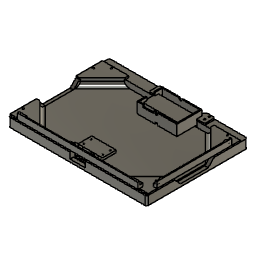
fusion_export (Autodesk Fusion 360 design; units mm, degrees)
Autodesk Fusion 360 part; units mm, degrees
note: some values were not read from the file. Chosen so that the rebuilt part matches the saved one: which face or edge a step refers to. Set by a fixed rule: which sketch regions a step uses.
sketch "Skizze1" plane through (0, 0, 0) normal (0, 0, 1) x (1, 0, 0)
  line L0 (88.5, 66) -> (-88.5, 66)
  line L1 (-90.5, 64) -> (-90.5, -64)
  line L2 (-88.5, -66) -> (88.5, -66)
  line L3 (90.5, -64) -> (90.5, 64)
  line L4 (90.5, 66) -> (-90.5, -66) construction
  line L5 (-90.5, 66) -> (90.5, -66) construction
  line L6 (-86, 52.5) -> (86, 52.5)
  line L7 (86, 52.5) -> (86, -59.5)
  line L8 (86, -59.5) -> (-86, -59.5)
  line L9 (-86, -59.5) -> (-86, 52.5)
  line L10 (0, 0) -> (0, 110) construction
  line L11 (-74, 48.5) -> (74, 48.5)
  line L12 (74, 48.5) -> (74, -48.5)
  line L13 (74, -48.5) -> (-74, -48.5)
  line L14 (-74, -48.5) -> (-74, 48.5)
  line L15 (0, 0) -> (180, 0) construction
  line L16 (-10, -59.5) -> (10, -59.5)
  line L17 (10, -59.5) -> (10, -66)
  line L18 (10, -66) -> (-10, -66)
  line L19 (-10, -66) -> (-10, -59.5)
  arc A0 (-90.5, -64) -> (-88.5, -66) centre (-88.5, -64) ccw
  arc A1 (88.5, -66) -> (90.5, -64) centre (88.5, -64) ccw
  arc A2 (-88.5, 66) -> (-90.5, 64) centre (-88.5, 64) ccw
  arc A3 (90.5, 64) -> (88.5, 66) centre (88.5, 64) ccw
  circle A4 centre (-12.5, -62) radius 0.9
  circle A5 centre (12.5, -62) radius 0.9
  line L20 (-20, -66) -> (-20, -59.5)
  line L21 (20, -59.5) -> (20, -66)
  circle A6 centre (-88, -49.5) radius 0.9
  circle A7 centre (-76, -61.5) radius 0.9
  line L22 (130, -3.5) -> (-113.5332, -3.5) construction
  line L23 (-86, -29.5) -> (-90.5, -29.5)
  line L24 (-56, -59.5) -> (-56, -66)
  line L25 (86, -29.5) -> (90.5, -29.5)
  circle A8 centre (88, -49.5) radius 0.9
  circle A9 centre (76, -61.5) radius 0.9
  line L26 (56, -59.5) -> (56, -66)
  line L27 (-86, 22.5) -> (-90.5, 22.5)
  circle A10 centre (-76, 54.5) radius 0.9
  line L28 (-56, 52.5) -> (-56, 59)
  line L29 (56, 52.5) -> (56, 59)
  line L30 (86, 22.5) -> (90.5, 22.5)
  circle A11 centre (76, 54.5) radius 0.9
  circle A12 centre (88, 42.5) radius 0.9
  circle A13 centre (-88, 42.5) radius 0.9
  line L31 (-56, 59) -> (-90.5, 59)
  line L32 (56, 59) -> (90.5, 59)
  line L33 (-56, 52.5) -> (-86, 22.5)
  line L34 (56, 52.5) -> (86, 22.5)
  line L35 (-86, -29.5) -> (-56, -59.5)
  line L36 (86, -29.5) -> (56, -59.5)
  line L37 (-56, -64) -> (-90.5, -64)
  line L38 (56, -64) -> (90.5, -64)
  line L39 (56, 57) -> (90.5, 57)
  line L40 (-56, 57) -> (-90.5, 57)
  line L41 (-13, 58) -> (36, 58)
  line L42 (36, 58) -> (36, 28)
  line L43 (36, 28) -> (-13, 28)
  line L44 (-13, 28) -> (-13, 58)
  line L45 (-14.5, 26.5) -> (-14.5, 59.5)
  line L46 (-14.5, 59.5) -> (37.5, 59.5)
  line L47 (37.5, 59.5) -> (37.5, 26.5)
  line L48 (37.5, 26.5) -> (-14.5, 26.5)
  line L49 (-7, 28) -> (7, 28)
  line L50 (7, 28) -> (7, 26.5)
  line L51 (7, 26.5) -> (-7, 26.5)
  line L52 (-7, 26.5) -> (-7, 28)
  line L53 (-14.5, 48) -> (-13, 48)
  line L54 (-13, 48) -> (-13, 38)
  line L55 (-13, 38) -> (-14.5, 38)
  line L56 (-14.5, 38) -> (-14.5, 48)
  line L57 (41, 43) -> (-35, 43) construction
  circle A14 centre (-20, 54.5) radius 0.9
  circle A15 centre (43, 54.5) radius 0.9
  line L58 (-25, 52.5) -> (-15, 52.5)
  line L59 (-15, 52.5) -> (-15, 66)
  line L60 (-15, 66) -> (-25, 66)
  line L61 (-25, 66) -> (-25, 52.5)
  line L62 (48, 52.5) -> (38, 52.5)
  line L63 (38, 52.5) -> (38, 66)
  line L64 (38, 66) -> (48, 66)
  line L65 (48, 66) -> (48, 52.5)
  line L66 (76, 54.5) -> (-76, 54.5) construction
  circle A16 centre (43, 57.5) radius 0.9
  circle A17 centre (-20, 57.5) radius 0.9
  circle A18 centre (43, 60.5) radius 0.9
  circle A19 centre (-20, 60.5) radius 0.9
  circle A20 centre (43, 63.5) radius 0.9
  circle A21 centre (-20, 63.5) radius 0.9
  line L67 (-16, -66) -> (16, -66)
  line L68 (16, -66) -> (16, -31.5)
  line L69 (16, -31.5) -> (-16, -31.5)
  line L70 (-16, -31.5) -> (-16, -66)
  line L71 (-16, -49.5) -> (16, -49.5)
  circle A22 centre (-12.5, -35.5) radius 0.9
  circle A23 centre (12.5, -35.5) radius 0.9
  circle A24 centre (-12.5, -45.5) radius 0.9
  circle A25 centre (12.5, -45.5) radius 0.9
  line L72 (-21, -40.5) -> (23, -40.5) construction
  line L73 (-10, -59.5) -> (-10, -49.5)
  line L74 (10, -59.5) -> (10, -49.5)
  line L75 (-15, 66) -> (-8.5, 59.5)
  line L76 (-15, 66) -> (-5.8076, 66) construction
  line L77 (38, 66) -> (31.5, 59.5)
  line L78 (-13, 53) -> (36, 53)
  line L79 (36, 53) -> (36, 33)
  line L80 (36, 33) -> (-13, 33)
  line L81 (-13, 33) -> (-13, 53)
  line L82 (-79, -66) -> (79, -66)
  line L83 (79, -66) -> (79, -63.5)
  line L84 (79, -63.5) -> (-79, -63.5)
  line L85 (-79, -63.5) -> (-79, -66)
  line L86 (-79, -63.5) -> (-73, -63.5)
  line L87 (-73, -63.5) -> (-73, -59.5)
  line L88 (-73, -59.5) -> (-79, -59.5)
  line L89 (-79, -59.5) -> (-79, -63.5)
  line L90 (73, -63.5) -> (73, -59.5)
  line L91 (79, -59.5) -> (79, -63.5)
  line L92 (90.5, -52.5) -> (88, -52.5)
  line L93 (88, -52.5) -> (88, 45.5)
  line L94 (88, 45.5) -> (90.5, 45.5)
  line L95 (90.5, 45.5) -> (90.5, -52.5)
  line L96 (88, -52.5) -> (86, -52.5)
  line L97 (86, -52.5) -> (86, -46.5)
  line L98 (86, -46.5) -> (88, -46.5)
  line L99 (88, -46.5) -> (88, -52.5)
  line L100 (88, 45.5) -> (86, 45.5)
  line L101 (86, 39.5) -> (88, 39.5)
  circle A26 centre (-88, -49.5) radius 1.25
  circle A27 centre (-76, -61.5) radius 1.25
  circle A28 centre (-12.5, -62) radius 1.25
  circle A29 centre (12.5, -62) radius 1.25
  circle A30 centre (76, -61.5) radius 1.25
  circle A31 centre (88, -49.5) radius 1.25
  circle A32 centre (88, 42.5) radius 1.25
  circle A33 centre (76, 54.5) radius 1.25
  circle A34 centre (-76, 54.5) radius 1.25
  circle A35 centre (-88, 42.5) radius 1.25
  circle A36 centre (43, 54.5) radius 1.25
  circle A37 centre (43, 57.5) radius 1.25
  circle A38 centre (43, 60.5) radius 1.25
  circle A39 centre (43, 63.5) radius 1.25
  circle A40 centre (-20, 54.5) radius 1.25
  circle A41 centre (-20, 57.5) radius 1.25
  circle A42 centre (-20, 60.5) radius 1.25
  circle A43 centre (-20, 63.5) radius 1.25
  line L102 (9, 26.5) -> (9, 28)
  line L103 (12, 26.5) -> (12, 28)
  line L104 (9, 58) -> (9, 59.5)
  line L105 (12, 58) -> (12, 59.5)
  line L106 (88, -46.5) -> (90.5, -46.5)
  line L107 (88, 39.5) -> (90.5, 39.5)
  dimension "d1" = 132
  dimension "d2" = 181
  dimension "d3" = 172
  dimension "d4" = 112
  dimension "d5" = 148
  dimension "d6" = 97
  dimension "d7" = 4
  dimension "d8" = 20
  dimension "d15" = 2
  dimension "d16" = 1.8
  dimension "d17" = 4
  dimension "d18" = 10
  dimension "d19" = 25
  dimension "d22" = 1.8
  dimension "d23" = 2
  dimension "d24" = 2
  dimension "d25" = 10
  dimension "d26" = 10
  dimension "d27" = 20
  dimension "d28" = 20
  dimension "d29" = 4.5
  dimension "d30" = 49
  dimension "d31" = 36
  dimension "d32" = -1.5
  dimension "d33" = 14
  dimension "d34" = 30
  dimension "d35" = 10
  dimension "d70" = 6
  dimension "d71" = 1.8
  dimension "d72" = 10
  dimension "d73" = 5
  dimension "d74" = 15
  dimension "d75" = 38
  dimension "d76" = 38
  dimension "d77" = 5
  dimension "d78" = 10
  dimension "d81" = 0
  dimension "d82" = 9
  dimension "d95" = 32
  dimension "d96" = 18
  dimension "d97" = 10
  dimension "d100" = 25
  dimension "d101" = -10
  dimension "d116" = 1.8
  dimension "d125" = 45
  dimension "d126" = 20
  dimension "d132" = 2.5
  dimension "d133" = 3
  dimension "d134" = 3
  dimension "d151" = 3
  dimension "d152" = 3
  dimension "d153" = 2.5
  dimension "d154" = 2.5
  dimension "d155" = 2
  dimension "d156" = 3
  constraint horizontal L0
  constraint perpendicular L0 L1
  constraint parallel L0 L2
  constraint parallel L1 L3
  constraint coincident L4 L10.start
  constraint coincident L5 L10.start
  constraint coincident L10.start L15.start
  constraint horizontal L6
  constraint vertical L7
  constraint horizontal L8
  constraint vertical L9
  constraint vertical L10
  constraint symmetric L7 L9 L10
  constraint horizontal L11
  constraint vertical L12
  constraint horizontal L13
  constraint vertical L14
  constraint symmetric L10 L12 L14
  constraint perpendicular L7 L15
  constraint symmetric L11 L13 L15
  constraint horizontal L16
  constraint vertical L17
  constraint horizontal L18
  constraint vertical L19
  constraint coincident L2 L17.end
  constraint coincident L8 L16.start
  constraint symmetric L10 L17 L19
  constraint coincident L4.end L1
  constraint coincident L4.end L2
  constraint tangent L1 A0
  constraint tangent L2 A0
  constraint coincident L5.end L3
  constraint coincident L5.end L2
  constraint tangent L3 A1
  constraint tangent L2 A1
  constraint equal A0 A1
  constraint coincident L5.start L0
  constraint coincident L5.start L1
  constraint tangent L0 A2
  constraint tangent L1 A2
  constraint equal A0 A2
  constraint coincident L4.start L0
  constraint coincident L4.start L3
  constraint tangent L0 A3
  constraint tangent L3 A3
  constraint equal A0 A3
  constraint equal A4 A5
  constraint symmetric L10 A4 A5
  constraint coincident L2 L20.start
  constraint coincident L8 L20.end
  constraint perpendicular L8 L20
  constraint coincident L8 L21.start
  constraint coincident L2 L21.end
  constraint perpendicular L2 L21
  constraint symmetric L10 L20 L21
  constraint equal A6 A7
  constraint perpendicular L14 L22
  constraint symmetric L6 L8 L22
  constraint coincident L9 L23.start
  constraint coincident L1 L23.end
  constraint perpendicular L1 L23
  constraint coincident L8 L24.start
  constraint coincident L2 L24.end
  constraint perpendicular L2 L24
  constraint symmetric L10 A6 A8
  constraint symmetric L10 A7 A9
  constraint symmetric L10 L23.start L25.start
  constraint symmetric L10 L23.end L25.end
  constraint symmetric L10 L24.start L26.start
  constraint symmetric L10 L24.end L26.end
  constraint symmetric A6 L22 A13
  constraint symmetric A7 L22 A10
  constraint symmetric L22 L23.start L27.start
  constraint symmetric L22 L23.end L27.end
  constraint symmetric L22 L24.start L28.start
  constraint symmetric L22 L24.end L28.end
  constraint symmetric L22 L25.start L30.start
  constraint symmetric L22 L25.end L30.end
  constraint symmetric L22 A8 A12
  constraint symmetric L22 A9 A11
  constraint symmetric L22 L26.start L29.start
  constraint symmetric L22 L26.end L29.end
  constraint coincident L1 L31.end
  constraint perpendicular L1 L31
  constraint coincident L3 L32.end
  constraint perpendicular L3 L32
  constraint coincident L24 L37.start
  constraint coincident L1 A0.start
  constraint horizontal L37
  constraint coincident L26 L38.start
  constraint coincident L3 A1.end
  constraint perpendicular L3 L38
  constraint collinear L37 L38
  constraint symmetric L22 L37.start L40.start
  constraint symmetric L22 L1.end L40.end
  constraint symmetric L22 L38.start L39.start
  constraint symmetric L22 L3.start L39.end
  constraint horizontal L41
  constraint vertical L42
  constraint horizontal L43
  constraint vertical L44
  constraint horizontal L49
  constraint vertical L50
  constraint horizontal L51
  constraint vertical L52
  constraint coincident L48 L50.end
  constraint coincident L43 L49.start
  constraint horizontal L53
  constraint vertical L54
  constraint horizontal L55
  constraint vertical L56
  constraint coincident L45 L53.start
  constraint perpendicular L42 L57
  constraint symmetric L46 L48 L57
  constraint symmetric L53 L55 L57
  constraint collinear L44 L54
  constraint equal A14 A15
  constraint horizontal L58
  constraint vertical L59
  constraint horizontal L60
  constraint vertical L61
  constraint coincident L0 L59.end
  constraint coincident L6 L58.start
  constraint horizontal L62
  constraint vertical L63
  constraint horizontal L64
  constraint vertical L65
  constraint coincident L0 L63.end
  constraint coincident L6 L62.start
  constraint coincident A11.centre L66.start
  constraint coincident A10.centre L66.end
  constraint coincident A14.centre L66
  constraint coincident A15.centre L66
  constraint horizontal L67
  constraint vertical L68
  constraint horizontal L69
  constraint vertical L70
  constraint coincident L2 L67.start
  constraint symmetric L10 L68 L70
  constraint coincident L68 L71.end
  constraint perpendicular L68 L71
  constraint symmetric L10 A22 A23
  constraint horizontal L72
  constraint symmetric A22 A24 L72
  constraint symmetric L69 L71 L72
  constraint coincident L71 L73.end
  constraint perpendicular L71 L73
  constraint coincident L71 L74.end
  constraint perpendicular L71 L74
  constraint horizontal L76
  constraint coincident L46 L75.end
  constraint coincident L46 L77.end
  constraint perpendicular L75 L77
  constraint horizontal L78
  constraint vertical L79
  constraint horizontal L80
  constraint vertical L81
  constraint coincident L42 L79.end
  constraint coincident L44 L78.start
  constraint symmetric L57 L78 L80
  constraint horizontal L82
  constraint vertical L83
  constraint horizontal L84
  constraint vertical L85
  constraint symmetric L10 L83 L85
  constraint collinear L2 L82
  constraint horizontal L86
  constraint vertical L87
  constraint horizontal L88
  constraint vertical L89
  constraint coincident L8 L87.end
  constraint symmetric L10 L84.end L83.end
  constraint symmetric L10 L86.end L90.start
  constraint symmetric L10 L87.end L90.end
  constraint symmetric L10 L88.end L91.start
  constraint horizontal L92
  constraint vertical L93
  constraint horizontal L94
  constraint vertical L95
  constraint coincident L3 L92.start
  constraint horizontal L96
  constraint vertical L97
  constraint horizontal L98
  constraint vertical L99
  constraint coincident L7 L97.end
  constraint symmetric L22 L92 L94
  constraint symmetric L22 L92.end L93.end
  constraint symmetric L22 L96.end L100.end
  constraint symmetric L22 L97.end L101.start
  constraint symmetric L22 L98.end L101.end
  constraint concentric A6 A26
  constraint concentric A7 A27
  constraint concentric A4 A28
  constraint concentric A5 A29
  constraint concentric A9 A30
  constraint concentric A8 A31
  constraint concentric A12 A32
  constraint concentric A11 A33
  constraint concentric A13 A35
  constraint concentric A15 A36
  constraint concentric A16 A37
  constraint concentric A18 A38
  constraint concentric A20 A39
  constraint concentric A14 A40
  constraint concentric A17 A41
  constraint concentric A19 A42
  constraint concentric A21 A43
  constraint equal A40 A41
  constraint equal A41 A42
  constraint equal A42 A43
  constraint equal A36 A43
  constraint equal A36 A37
  constraint equal A37 A38
  constraint equal A38 A39
  constraint equal A33 A39
  constraint equal A32 A33
  constraint equal A32 A34
  constraint equal A34 A35
  constraint equal A31 A35
  constraint equal A30 A31
  constraint equal A29 A30
  constraint equal A28 A29
  constraint equal A27 A28
  constraint equal A26 A27
  constraint coincident L48 L102.start
  constraint coincident L43 L102.end
  constraint coincident L48 L103.start
  constraint coincident L43 L103.end
  constraint vertical L102
  constraint vertical L103
  constraint coincident L41 L104.start
  constraint coincident L46 L104.end
  constraint perpendicular L46 L104
  constraint coincident L41 L105.start
  constraint coincident L46 L105.end
  constraint perpendicular L46 L105
  constraint collinear L102 L104
  constraint collinear L103 L105
  constraint coincident L3 L106.end
  constraint collinear L98 L106
  constraint coincident L3 L107.end
  constraint collinear L101 L107
  measures "d1" distance of L5.start L4.end
  measures "d2" distance of L4.end L5.end
  measures "d3" distance of L6.start L6.end
  measures "d4" distance of L6.start L8.end
  measures "d5" distance of L11.start L11.end
  measures "d6" distance of L11.start L13.end
  measures "d7" distance of L6 L11
  measures "d8" distance of L17 L19
  measures "d15" radius of A0
  measures "d16" diameter of A4
  measures "d17" distance of L2 A4.centre
  measures "d18" distance of L19 L20
  measures "d19" distance of A4.centre A5.centre
  measures "d22" diameter of A6
  measures "d23" distance of L9 A6.centre
  measures "d24" distance of L8 A7.centre
  measures "d25" distance of L8 A6.centre
  measures "d26" distance of L9 A7.centre
  measures "d27" distance of A6.centre L23
  measures "d28" distance of A7.centre L24
  measures "d29" distance of L8 L37
  measures "d30" distance of L41.start L41.end
  measures "d31" distance of L10 L42
  measures "d33" distance of L50 L52
  measures "d34" distance of L41 L43
  measures "d35" distance of L53.start L55.end
  measures "d70" distance of L44 L52
  measures "d71" diameter of A14
  measures "d72" distance of L59 L61
  measures "d73" distance of A14.centre L59
  measures "d74" distance of L10 L59
  measures "d75" distance of L0 L43
  measures "d76" distance of L10 L63
  measures "d77" distance of A15.centre L63
  measures "d78" distance of L63 L65
  measures "d95" distance of L68 L70
  measures "d96" distance of L69 L71
  measures "d97" distance of L8 L71
  measures "d116" diameter of A22
  measures "d125" angle of L75 L76
  measures "d126" distance of L78 L80
  measures "d132" distance of L82 L84
  measures "d133" distance of A7.centre L85
  measures "d134" distance of A7.centre L87
  measures "d143" diameter of L8.end
  measures "d151" distance of A8.centre L92
  measures "d152" distance of A8.centre L98
  measures "d153" distance of L3 L93
  measures "d154" diameter of A26
  measures "d155" distance of L50 L102
  measures "d156" distance of L102 L103
extrude "Extrusion1" add sketch "Skizze1" against normal blind 1.5 contours L0 L3 L6 A3 L29 L32 L65 | L0 L6 L62 L63 L64 L65 | L0 L46 L75 L77 | L6 L46 L47 L63 L77 | L6 L11 L34 L47 L62 | L3 L29 L32 L39 | L0 L6 L58 L59 L60 L61 | L6 L45 L46 L59 L75 | L6 L41 L42 L46 L47 L79 L105 | L3 L6 L7 L29 L39 L94 L100 | L6 L7 L11 L12 L34 | L0 L1 L6 A2 L28 L31 L61 | L6 L11 L33 L45 L58 | L6 L41 L44 L45 L46 L81 L104 | L6 L11 L42 L47 L79 | L41 L46 L104 L105 | L3 L93 L94 L95 A32 L107 | L6 L11 L44 L45 L81 | L6 L11 L42 L44 L79 L81 | L6 L42 L44 L78 L79 L81 | L41 L42 L44 L78 | L7 L93 L100 L101 A32 | L7 L12 L34 L36 | L3 L30 L93 L95 L107 | L6 L9 L11 L14 L33 | L1 L6 L9 L27 L28 L40 | L7 L30 L93 L101 | L7 L8 L12 L13 L36 L97 | L7 L25 L30 L93 | L3 L25 L30 L93 L95 | A12 L93 A32 | A12 L93 A32 | L1 L28 L31 L40 | L7 L25 L93 L98 | L8 L13 L36 L68 | L3 L25 L93 L95 L106 | A12 L93 | A12 L93 | L9 L14 L33 L35 | L1 L9 L23 L27 | L7 L93 L96 L97 L98 L99 A31 | L13 L68 L70 L71 | L8 L21 L26 L84 | L8 L26 L84 L90 | L3 L92 L93 L95 L99 A31 L106 | L8 L9 L13 L14 L35 L88 | L1 L8 L9 L23 L37 L85 L89 | L3 L7 L8 L38 L83 L91 L92 L96 | L8 L13 L35 L70 | L8 L68 L71 L74 | L8 L84 L90 L91 | L8 L21 L68 L84 | L26 L38 L83 L84 | L2 L21 L26 L82 L84 | A8 L93 L99 A31 | A8 L93 L99 A31 | L8 L70 L71 L73 | L8 L17 L68 L84 | L8 L16 L71 L73 L74 | L2 L21 L68 L82 L84 | L2 L26 L38 L82 L83 | L2 A1 L38 L83 | L2 A0 L37 L85 | L8 L84 L86 L87 L88 L89 | L8 L24 L84 L87 | L8 L20 L24 L84 | A8 L93 L99 | A8 L93 L99 | L8 L20 L70 L84 | L8 L19 L70 L84 | L8 L16 L17 L19 L84 | L2 L17 L67 L68 L82 L84 | L24 L37 L84 L85 L86 | L2 L24 L37 L82 L85 | L2 L20 L24 L82 L84 | L2 L19 L67 L70 L82 L84 | L2 L20 L70 L82 L84 | L2 L17 L18 L19 L67 L82 L84 | A4 | A5 | A6 | A7 | A9 | A10 | A11 | A13 | A14 | A15 | A16 | A17 | A18 | A19 | A20 | A21 | A26 | A27 | A28 | A29 | A30 | A33 | A34 | A35 | A36 | A37 | A38 | A39 | A40 | A41 | A42 | A43 makes body 1
extrude "Extrusion2" add sketch "Skizze1" along normal blind 2 contours L0 L3 L6 A3 L29 L32 L65 | L0 L6 L62 L63 L64 L65 | L0 L46 L75 L77 | L6 L46 L47 L63 L77 | L3 L29 L32 L39 | L0 L6 L58 L59 L60 L61 | L6 L45 L46 L59 L75 | L6 L41 L42 L46 L47 L79 L105 | L3 L6 L7 L29 L39 L94 L100 | L0 L1 L6 A2 L28 L31 L61 | L6 L41 L44 L45 L46 L81 L104 | L41 L46 L104 L105 | L3 L93 L94 L95 A32 L107 | L6 L42 L44 L78 L79 L81 | L41 L42 L44 L78 | L7 L93 L100 L101 A32 | L3 L30 L93 L95 L107 | L1 L6 L9 L27 L28 L40 | L7 L30 L93 L101 | L7 L25 L30 L93 | L3 L25 L30 L93 L95 | A12 L93 A32 | A12 L93 A32 | L1 L28 L31 L40 | L7 L25 L93 L98 | L3 L25 L93 L95 L106 | A12 L93 | A12 L93 | L1 L9 L23 L27 | L7 L93 L96 L97 L98 L99 A31 | L8 L21 L26 L84 | L8 L26 L84 L90 | L3 L92 L93 L95 L99 A31 L106 | L1 L8 L9 L23 L37 L85 L89 | L3 L7 L8 L38 L83 L91 L92 L96 | L8 L84 L90 L91 | L8 L21 L68 L84 | L26 L38 L83 L84 | L2 L21 L26 L82 L84 | A8 L93 L99 A31 | A8 L93 L99 A31 | L8 L17 L68 L84 | L2 L21 L68 L82 L84 | L2 L26 L38 L82 L83 | L2 A1 L38 L83 | L2 A0 L37 L85 | L8 L84 L86 L87 L88 L89 | L8 L24 L84 L87 | L8 L20 L24 L84 | A8 L93 L99 | A8 L93 L99 | L8 L20 L70 L84 | L8 L19 L70 L84 | L8 L16 L17 L19 L84 | L2 L17 L67 L68 L82 L84 | L24 L37 L84 L85 L86 | L2 L24 L37 L82 L85 | L2 L20 L24 L82 L84 | L2 L19 L67 L70 L82 L84 | L2 L20 L70 L82 L84 | L2 L17 L18 L19 L67 L82 L84 | A4 | A5 | A6 | A7 | A9 | A10 | A11 | A13 | A14 | A15 | A16 | A17 | A18 | A19 | A20 | A21 | A26 | A27 | A28 | A29 | A30 | A33 | A34 | A35 | A36 | A37 | A38 | A39 | A40 | A41 | A42 | A43 bodies 1
chamfer "Fase1" distance 1 distance2 1 4 edges at (0, -48.5, -1.5) (74, 0, -1.5) (0, 48.5, -1.5) (-74, 0, -1.5) measured on face at (24.6667, -60.1667, -1.5) measured on face at (24.6667, -60.1667, -1.5) measured on face at (24.6667, -60.1667, -1.5) measured on face at (24.6667, -60.1667, -1.5) on bodies 1
extrude "Extrusion3" add sketch "Skizze1" along normal blind 10 contours L0 L3 L6 A3 L29 L32 L65 | L0 L6 L62 L63 L64 L65 | L3 L29 L32 L39 | L0 L6 L58 L59 L60 L61 | L3 L6 L7 L29 L39 L94 L100 | L0 L1 L6 A2 L28 L31 L61 | L3 L93 L94 L95 A32 L107 | L7 L93 L100 L101 A32 | L3 L30 L93 L95 L107 | L1 L6 L9 L27 L28 L40 | L7 L30 L93 L101 | A12 L93 A32 | A12 L93 A32 | L1 L28 L31 L40 | L7 L25 L93 L98 | L3 L25 L93 L95 L106 | L7 L93 L96 L97 L98 L99 A31 | L8 L21 L26 L84 | L8 L26 L84 L90 | L3 L92 L93 L95 L99 A31 L106 | L1 L8 L9 L23 L37 L85 L89 | L3 L7 L8 L38 L83 L91 L92 L96 | L8 L84 L90 L91 | L8 L21 L68 L84 | L26 L38 L83 L84 | L2 L21 L26 L82 L84 | A8 L93 L99 A31 | A8 L93 L99 A31 | L8 L17 L68 L84 | L2 L21 L68 L82 L84 | L2 L26 L38 L82 L83 | L2 A1 L38 L83 | L2 A0 L37 L85 | L8 L84 L86 L87 L88 L89 | L8 L24 L84 L87 | L8 L20 L24 L84 | L8 L20 L70 L84 | L8 L19 L70 L84 | L2 L17 L67 L68 L82 L84 | L24 L37 L84 L85 L86 | L2 L24 L37 L82 L85 | L2 L20 L24 L82 L84 | L2 L19 L67 L70 L82 L84 | L2 L20 L70 L82 L84 | A26 | A27 | A28 | A29 | A30 | A33 | A34 | A35 | A36 | A37 | A38 | A39 | A40 | A41 | A42 | A43 bodies 1
extrude "Extrusion4" add sketch "Skizze1" along normal blind 10 and the other way blind -1 separate body contours L6 L7 L11 L12 L34 | L11 L12 L34 | L6 L9 L11 L14 L33 | L7 L8 L12 L13 L36 L97 | L12 L13 L36 | L11 L14 L33 | L8 L9 L13 L14 L35 L88 | L13 L14 L35 makes body 2 at (76, -49.5, 1) makes body 3 at (-76, 42.5, 1) makes body 4 at (-76, -49.5, 1) makes body 5 at (76, 42.5, 1)
extrude "Extrusion5" add sketch "Skizze1" along normal blind 12 and the other way blind -10 contours L3 L6 L7 L29 L39 L94 L100 | L6 L7 L11 L12 L34 | L11 L12 L34 | L3 L93 L94 L95 A32 L107 | L7 L93 L100 L101 A32 | L3 L30 L93 L95 L107 | L6 L9 L11 L14 L33 | L1 L6 L9 L27 L28 L40 | L7 L30 L93 L101 | L7 L8 L12 L13 L36 L97 | L12 L13 L36 | L11 L14 L33 | L7 L25 L93 L98 | L3 L25 L93 L95 L106 | L7 L93 L96 L97 L98 L99 A31 | L8 L26 L84 L90 | L3 L92 L93 L95 L99 A31 L106 | L8 L9 L13 L14 L35 L88 | L1 L8 L9 L23 L37 L85 L89 | L13 L14 L35 | L3 L7 L8 L38 L83 L91 L92 L96 | L8 L84 L90 L91 | L26 L38 L83 L84 | L8 L84 L86 L87 L88 L89 | L8 L24 L84 L87 | L24 L37 L84 L85 L86 bodies 2 3 4 5
extrude "Extrusion6" add sketch "Skizze1" along normal blind 1 and the other way blind -3 contours L6 L11 L34 L47 L62 | L6 L11 L33 L45 L58 | L6 L11 L42 L47 L79 | L11 L12 L13 L14 L33 L34 L35 L36 L45 L47 L48 L51 L56 L68 L69 L70 | L6 L11 L44 L45 L81 | L6 L11 L42 L44 L79 L81 | L11 L42 L43 L47 L48 L79 L103 | L7 L12 L34 L36 | L11 L44 L45 L53 L81 | L11 L42 L44 L54 L79 L80 L81 | L12 L13 L36 | L44 L45 L53 L54 L55 L56 L81 | L42 L43 L44 L49 L80 | L43 L48 L102 L103 | L8 L13 L36 L68 | L9 L14 L33 L35 | L43 L44 L45 L48 L52 L55 L81 | L43 L48 L50 L102 | L13 L68 L70 L71 | L13 L68 L69 L70 | L8 L9 L13 L14 L35 L88 | L13 L14 L35 | L43 L48 L49 L50 L51 L52 | L8 L13 L35 L70 | L8 L68 L71 L74 | L8 L70 L71 L73 | L8 L16 L71 L73 L74 | A22 | A23 | A24 | A25 bodies 2 3 4 5
move_face "Flächen versetzen1" offset -0.5 4 faces at (76, -59.5, 4.6667) (86, 42.5, 4.6667) (-86, -49.5, 4.6667) (-76, 52.5, 4.6667) on bodies 2
fillet "Abrundung1" radius 1 4 edges at (85.5, -59, 5.5) (-85.5, 52, 5.5) (-85.5, -59, 5.5) (85.5, 52, 5.5) on bodies 2
fillet "Abrundung2" radius 5 4 edges at (-71, 37.5, 3) (71, 37.5, 3) (-71, -44.5, 3) (71, -44.5, 3) on bodies 2
extrude "Extrusion8" add sketch "Skizze1" along normal blind 6.5 and the other way blind -5 separate body contours L6 L41 L42 L46 L47 L79 L105 | L6 L41 L44 L45 L46 L81 L104 | L6 L11 L42 L47 L79 | L41 L46 L104 L105 | L6 L11 L44 L45 L81 | L6 L11 L42 L44 L79 L81 | L6 L42 L44 L78 L79 L81 | L11 L42 L43 L47 L48 L79 L103 | L41 L42 L44 L78 | L11 L44 L45 L53 L81 | L11 L42 L44 L54 L79 L80 L81 | L44 L45 L53 L54 L55 L56 L81 | L42 L43 L44 L49 L80 | L43 L48 L102 L103 | L43 L44 L45 L48 L52 L55 L81 | L43 L48 L50 L102 | L43 L48 L49 L50 L51 L52 makes body 6
extrude "Extrusion9" add sketch "Skizze1" along normal blind 19 and the other way blind -6.5 contours L6 L41 L42 L46 L47 L79 L105 | L6 L41 L44 L45 L46 L81 L104 | L6 L11 L42 L47 L79 | L41 L46 L104 L105 | L6 L11 L44 L45 L81 | L11 L42 L43 L47 L48 L79 L103 | L11 L44 L45 L53 L81 | L44 L45 L53 L54 L55 L56 L81 | L43 L48 L102 L103 | L43 L44 L45 L48 L52 L55 L81 | L43 L48 L50 L102 | L43 L48 L49 L50 L51 L52 bodies 6
extrude "Extrusion10" add sketch "Skizze1" along normal blind 12 and the other way blind -10 contours L0 L6 L62 L63 L64 L65 | L6 L46 L47 L63 L77 | L0 L6 L58 L59 L60 L61 | L6 L45 L46 L59 L75 | A14 | A15 | A18 | A19 | A36 | A38 | A40 | A42 bodies 6
chamfer "Fase3" distance 8 distance2 8 4 edges at (-88.25, 22.5, 2) (88.25, 22.5, 2) (-88.25, -29.5, 2) (88.25, -29.5, 2) measured on face at (-87.5, 5.1667, 2) measured on face at (87.5, 5.1667, 2) measured on face at (-87.5, 5.1667, 2) measured on face at (87.5, 5.1667, 2) on bodies 1
chamfer "Fase4" distance 2 distance2 2 1 edges at (0, -59.5, 2) measured on face at (-3.3333, -63.8333, 2) on bodies 1
extrude "Extrusion11" cut sketch "Skizze1" along normal blind 22 and the other way blind -16 contours L43 L48 L49 L50 L51 L52 bodies 6
extrude "Extrusion12" add sketch "Skizze1" along normal blind 12 and the other way blind -10 separate body contours L8 L68 L71 L74 | L8 L70 L71 L73 | L8 L17 L68 L84 | L8 L19 L70 L84 | L2 L17 L67 L68 L82 L84 | L2 L19 L67 L70 L82 L84 makes body 7 at (-12.8645, -53.2512, 10) makes body 8 at (12.8645, -53.2512, 10)
extrude "Extrusion13" add sketch "Skizze1" along normal blind 8 and the other way blind -5 separate body contours L13 L68 L70 L71 | L13 L68 L69 L70 makes body 9
extrude "Extrusion14" add sketch "Skizze1" along normal blind 10 and the other way blind -5 contours L8 L68 L71 L74 | L8 L70 L71 L73 bodies 7 8 9
move_face "Flächen versetzen2" offset -0.5 2 faces at (-12, -59.5, 6.6667) (14, -59.5, 6.6667) on bodies 7
chamfer "Fase6" distance 4 angle 45 2 edges at (13, -49.5, 12) (-13, -49.5, 12) on bodies 7
extrude "Extrusion15" cut sketch "Skizze1" along normal blind 19 and the other way blind -15 contours L11 L44 L45 L53 L81 | L44 L45 L53 L54 L55 L56 L81 bodies 6
extrude "Extrusion16" add sketch "Skizze1" along normal blind 15 and the other way blind -5 contours L6 L11 L42 L44 L79 L81 | L6 L42 L44 L78 L79 L81 | L11 L42 L44 L54 L79 L80 L81 bodies 6
extrude "Extrusion17" add sketch "Skizze1" along normal blind 20 and the other way blind -12 separate body contours L3 L93 L94 L95 A32 L107 | L3 L30 L93 L95 L107 | L3 L25 L30 L93 L95 | L3 L25 L93 L95 L106 | L3 L92 L93 L95 L99 A31 L106 | L26 L38 L83 L84 | L2 L21 L26 L82 L84 | L2 L21 L68 L82 L84 | L2 L26 L38 L82 L83 | L2 L17 L67 L68 L82 L84 | L24 L37 L84 L85 L86 | L2 L24 L37 L82 L85 | L2 L20 L24 L82 L84 | L2 L19 L67 L70 L82 L84 | L2 L20 L70 L82 L84 | L2 L17 L18 L19 L67 L82 L84 makes body 10 at (26.3333, -63.5, 17.3333) makes body 11 at (90.5, -19.8333, 17.3333)
sketch "Skizze2" plane through (0, 0, 20) normal (0, 0, 1) x (-1, 0, 0)
  line L0 (73, 16) -> (79, 16)
  line L1 (79, 16) -> (79, 20)
  line L2 (79, 20) -> (-79, 20)
  line L3 (-79, 20) -> (-79, 16)
  line L4 (-79, 16) -> (-73, 16)
  line L5 (-73, 16) -> (-73, 13)
  line L6 (-73, 13) -> (73, 13)
  line L7 (73, 13) -> (73, 16)
  line L8 (79, 66) -> (-79, 66)
  line L9 (-79, 66) -> (-79, 63.5)
  line L10 (-79, 63.5) -> (79, 63.5)
  line L11 (79, 63.5) -> (79, 66)
  circle A0 centre (-70, 63.5) radius 1.25
  line L12 (0, 0) -> (0, 97.9968) construction
  circle A1 centre (-67.971, 63.5) radius 1.25
  circle A2 centre (-65.942, 63.5) radius 1.25
  circle A3 centre (-63.913, 63.5) radius 1.25
  circle A4 centre (-61.8841, 63.5) radius 1.25
  circle A5 centre (-59.8551, 63.5) radius 1.25
  circle A6 centre (-57.8261, 63.5) radius 1.25
  circle A7 centre (-55.7971, 63.5) radius 1.25
  circle A8 centre (-53.7681, 63.5) radius 1.25
  circle A9 centre (-51.7391, 63.5) radius 1.25
  circle A10 centre (-49.7101, 63.5) radius 1.25
  circle A11 centre (-47.6812, 63.5) radius 1.25
  circle A12 centre (-45.6522, 63.5) radius 1.25
  circle A13 centre (-43.6232, 63.5) radius 1.25
  circle A14 centre (-41.5942, 63.5) radius 1.25
  circle A15 centre (-39.5652, 63.5) radius 1.25
  circle A16 centre (-37.5362, 63.5) radius 1.25
  circle A17 centre (-35.5072, 63.5) radius 1.25
  circle A18 centre (-33.4783, 63.5) radius 1.25
  circle A19 centre (-31.4493, 63.5) radius 1.25
  circle A20 centre (-29.4203, 63.5) radius 1.25
  circle A21 centre (-27.3913, 63.5) radius 1.25
  circle A22 centre (-25.3623, 63.5) radius 1.25
  circle A23 centre (-23.3333, 63.5) radius 1.25
  circle A24 centre (-21.3043, 63.5) radius 1.25
  circle A25 centre (-19.2754, 63.5) radius 1.25
  circle A26 centre (-17.2464, 63.5) radius 1.25
  circle A27 centre (-15.2174, 63.5) radius 1.25
  circle A28 centre (-13.1884, 63.5) radius 1.25
  circle A29 centre (-11.1594, 63.5) radius 1.25
  circle A30 centre (-9.1304, 63.5) radius 1.25
  circle A31 centre (-7.1014, 63.5) radius 1.25
  circle A32 centre (-5.0725, 63.5) radius 1.25
  circle A33 centre (-3.0435, 63.5) radius 1.25
  circle A34 centre (-1.0145, 63.5) radius 1.25
  circle A35 centre (1.0145, 63.5) radius 1.25
  circle A36 centre (3.0435, 63.5) radius 1.25
  circle A37 centre (5.0725, 63.5) radius 1.25
  circle A38 centre (7.1014, 63.5) radius 1.25
  circle A39 centre (9.1304, 63.5) radius 1.25
  circle A40 centre (11.1594, 63.5) radius 1.25
  circle A41 centre (13.1884, 63.5) radius 1.25
  circle A42 centre (15.2174, 63.5) radius 1.25
  circle A43 centre (17.2464, 63.5) radius 1.25
  circle A44 centre (19.2754, 63.5) radius 1.25
  circle A45 centre (21.3043, 63.5) radius 1.25
  circle A46 centre (23.3333, 63.5) radius 1.25
  circle A47 centre (25.3623, 63.5) radius 1.25
  circle A48 centre (27.3913, 63.5) radius 1.25
  circle A49 centre (29.4203, 63.5) radius 1.25
  circle A50 centre (31.4493, 63.5) radius 1.25
  circle A51 centre (33.4783, 63.5) radius 1.25
  circle A52 centre (35.5072, 63.5) radius 1.25
  circle A53 centre (37.5362, 63.5) radius 1.25
  circle A54 centre (39.5652, 63.5) radius 1.25
  circle A55 centre (41.5942, 63.5) radius 1.25
  circle A56 centre (43.6232, 63.5) radius 1.25
  circle A57 centre (45.6522, 63.5) radius 1.25
  circle A58 centre (47.6812, 63.5) radius 1.25
  circle A59 centre (49.7101, 63.5) radius 1.25
  circle A60 centre (51.7391, 63.5) radius 1.25
  circle A61 centre (53.7681, 63.5) radius 1.25
  circle A62 centre (55.7971, 63.5) radius 1.25
  circle A63 centre (57.8261, 63.5) radius 1.25
  circle A64 centre (59.8551, 63.5) radius 1.25
  circle A65 centre (61.8841, 63.5) radius 1.25
  circle A66 centre (63.913, 63.5) radius 1.25
  circle A67 centre (65.942, 63.5) radius 1.25
  circle A68 centre (67.971, 63.5) radius 1.25
  circle A69 centre (70, 63.5) radius 1.25
  dimension "d143" = 2.5
  dimension "d144" = 70
  dimension "d147" = 140
  dimension "d148" = 0
  constraint coincident L10 A0.centre
  constraint coincident L12.start origin
  constraint perpendicular L2 L12
  measures "d143" diameter of A0
  measures "d144" distance of A0.centre L12
extrude "Extrusion19" cut sketch "Skizze2" against normal blind 8 contours L10 A68 A69 | L10 A68 A69 | L10 A0 A1 | L10 A0 A1 | L10 A68 A69 | L10 A68 A69 | L10 A67 A68 A69 | L10 A67 A68 A69 | L10 A0 A1 | L10 A0 A1 | L10 A0 A1 A2 | L10 A0 A1 A2 | L10 A66 A67 A68 | L10 A67 A68 | L10 A67 A68 | L10 A66 A67 A68 | L10 A1 A2 A3 | L10 A1 A2 | L10 A1 A2 | L10 A1 A2 A3 | L10 A65 A66 A67 | L10 A66 A67 | L10 A66 A67 | L10 A65 A66 A67 | L10 A2 A3 A4 | L10 A2 A3 | L10 A2 A3 | L10 A2 A3 A4 | L10 A64 A65 A66 | L10 A65 A66 | L10 A65 A66 | L10 A64 A65 A66 | L10 A3 A4 A5 | L10 A3 A4 | L10 A3 A4 | L10 A3 A4 A5 | L10 A63 A64 A65 | L10 A64 A65 | L10 A64 A65 | L10 A63 A64 A65 | L10 A4 A5 A6 | L10 A4 A5 | L10 A4 A5 | L10 A4 A5 A6 | L10 A62 A63 A64 | L10 A63 A64 | L10 A63 A64 | L10 A62 A63 A64 | L10 A5 A6 A7 | L10 A5 A6 | L10 A5 A6 | L10 A5 A6 A7 | L10 A61 A62 A63 | L10 A62 A63 | L10 A62 A63 | L10 A61 A62 A63 | L10 A6 A7 A8 | L10 A6 A7 | L10 A6 A7 | L10 A6 A7 A8 | L10 A60 A61 A62 | L10 A61 A62 | L10 A61 A62 | L10 A60 A61 A62 | L10 A7 A8 A9 | L10 A7 A8 | L10 A7 A8 | L10 A7 A8 A9 | L10 A59 A60 A61 | L10 A60 A61 | L10 A60 A61 | L10 A59 A60 A61 | L10 A8 A9 A10 | L10 A8 A9 | L10 A8 A9 | L10 A8 A9 A10 | L10 A58 A59 A60 | L10 A59 A60 | L10 A59 A60 | L10 A58 A59 A60 | L10 A9 A10 A11 | L10 A9 A10 | L10 A9 A10 | L10 A9 A10 A11 | L10 A57 A58 A59 | L10 A58 A59 | L10 A58 A59 | L10 A57 A58 A59 | L10 A10 A11 A12 | L10 A10 A11 | L10 A10 A11 | L10 A10 A11 A12 | L10 A56 A57 A58 | L10 A57 A58 | L10 A57 A58 | L10 A56 A57 A58 | L10 A11 A12 A13 | L10 A11 A12 | L10 A11 A12 | L10 A11 A12 A13 | L10 A55 A56 A57 | L10 A56 A57 | L10 A56 A57 | L10 A55 A56 A57 | L10 A12 A13 A14 | L10 A12 A13 | L10 A12 A13 | L10 A12 A13 A14 | L10 A54 A55 A56 | L10 A55 A56 | L10 A55 A56 | L10 A54 A55 A56 | L10 A13 A14 A15 | L10 A13 A14 | L10 A13 A14 | L10 A13 A14 A15 | L10 A53 A54 A55 | L10 A54 A55 | L10 A54 A55 | L10 A53 A54 A55 | L10 A14 A15 A16 | L10 A14 A15 | L10 A14 A15 | L10 A14 A15 A16 | L10 A52 A53 A54 | L10 A53 A54 | L10 A53 A54 | L10 A52 A53 A54 | L10 A15 A16 A17 | L10 A15 A16 | L10 A15 A16 | L10 A15 A16 A17 | L10 A51 A52 A53 | L10 A52 A53 | L10 A52 A53 | L10 A51 A52 A53 | L10 A16 A17 A18 | L10 A16 A17 | L10 A16 A17 | L10 A16 A17 A18 | L10 A50 A51 A52 | L10 A51 A52 | L10 A51 A52 | L10 A50 A51 A52 | L10 A17 A18 A19 | L10 A17 A18 | L10 A17 A18 | L10 A17 A18 A19 | L10 A49 A50 A51 | L10 A50 A51 | L10 A50 A51 | L10 A49 A50 A51 | L10 A18 A19 A20 | L10 A18 A19 | L10 A18 A19 | L10 A18 A19 A20 | L10 A48 A49 A50 | L10 A49 A50 | L10 A49 A50 | L10 A48 A49 A50 | L10 A19 A20 A21 | L10 A19 A20 | L10 A19 A20 | L10 A19 A20 A21 | L10 A47 A48 A49 | L10 A48 A49 | L10 A48 A49 | L10 A47 A48 A49 | L10 A20 A21 A22 | L10 A20 A21 | L10 A20 A21 | L10 A20 A21 A22 | L10 A46 A47 A48 | L10 A47 A48 | L10 A47 A48 | L10 A46 A47 A48 | L10 A21 A22 A23 | L10 A21 A22 | L10 A21 A22 | L10 A21 A22 A23 | L10 A45 A46 A47 | L10 A46 A47 | L10 A46 A47 | L10 A45 A46 A47 | L10 A22 A23 A24 | L10 A22 A23 | L10 A22 A23 | L10 A22 A23 A24 | L10 A44 A45 A46 | L10 A45 A46 | L10 A45 A46 | L10 A44 A45 A46 | L10 A23 A24 A25 | L10 A23 A24 | L10 A23 A24 | L10 A23 A24 A25 | L10 A43 A44 A45 | L10 A44 A45 | L10 A44 A45 | L10 A43 A44 A45 | L10 A24 A25 A26 | L10 A24 A25 | L10 A24 A25 | L10 A24 A25 A26 | L10 A42 A43 A44 | L10 A43 A44 | L10 A43 A44 | L10 A42 A43 A44 | L10 A25 A26 A27 | L10 A25 A26 | L10 A25 A26 | L10 A25 A26 A27 | L10 A41 A42 A43 | L10 A42 A43 | L10 A42 A43 | L10 A41 A42 A43 | L10 A26 A27 A28 | L10 A26 A27 | L10 A26 A27 | L10 A26 A27 A28 | L10 A40 A41 A42 | L10 A41 A42 | L10 A41 A42 | L10 A40 A41 A42 | L10 A27 A28 A29 | L10 A27 A28 | L10 A27 A28 | L10 A27 A28 A29 | L10 A39 A40 A41 | L10 A40 A41 | L10 A40 A41 | L10 A39 A40 A41 | L10 A28 A29 A30 | L10 A28 A29 | L10 A28 A29 | L10 A28 A29 A30 | L10 A38 A39 A40 | L10 A39 A40 | L10 A39 A40 | L10 A38 A39 A40 | L10 A29 A30 A31 | L10 A29 A30 | L10 A29 A30 | L10 A29 A30 A31 | L10 A37 A38 A39 | L10 A38 A39 | L10 A38 A39 | L10 A37 A38 A39 | L10 A30 A31 A32 | L10 A30 A31 | L10 A30 A31 | L10 A30 A31 A32 | L10 A36 A37 A38 | L10 A37 A38 | L10 A37 A38 | L10 A36 A37 A38 | L10 A31 A32 A33 | L10 A31 A32 | L10 A31 A32 | L10 A31 A32 A33 | L10 A35 A36 A37 | L10 A36 A37 | L10 A36 A37 | L10 A35 A36 A37 | L10 A32 A33 A34 | L10 A32 A33 | L10 A32 A33 | L10 A32 A33 A34 | L10 A34 A35 A36 | L10 A35 A36 | L10 A35 A36 | L10 A34 A35 A36 | L10 A33 A34 A35 | L10 A33 A34 | L10 A33 A34 | L10 A33 A34 A35 | L10 A34 A35 | L10 A34 A35 bodies 10
sketch "Skizze3" plane through (0, 0, 20) normal (0, 0, 1) x (-1, 0, 0)
  line L0 (-88, -41.25) -> (-88, 48.25)
  arc A0 (-88, 50.75) -> (-88, 48.25) centre (-88, 49.5) ccw
  line L1 (-88, 50.75) -> (-88, 52.5)
  line L2 (-88, 52.5) -> (-90.5, 52.5)
  line L3 (-90.5, 52.5) -> (-90.5, -45.5)
  line L4 (-90.5, -45.5) -> (-88, -45.5)
  line L5 (-88, -45.5) -> (-88, -43.75)
  arc A1 (-88, -41.25) -> (-88, -43.75) centre (-88, -42.5) ccw
  circle A2 centre (-88, -42.5) radius 2
  circle A3 centre (-88, 49.5) radius 2
  circle A4 centre (-88, -36.5) radius 1.25
  line L6 (-130, 3.5) -> (113.5332, 3.5)
  circle A5 centre (-88, -34.4487) radius 1.25
  circle A6 centre (-88, -32.3974) radius 1.25
  circle A7 centre (-88, -30.3462) radius 1.25
  circle A8 centre (-88, -28.2949) radius 1.25
  circle A9 centre (-88, -26.2436) radius 1.25
  circle A10 centre (-88, -24.1923) radius 1.25
  circle A11 centre (-88, -22.141) radius 1.25
  circle A12 centre (-88, -20.0897) radius 1.25
  circle A13 centre (-88, -18.0385) radius 1.25
  circle A14 centre (-88, -15.9872) radius 1.25
  circle A15 centre (-88, -13.9359) radius 1.25
  circle A16 centre (-88, -11.8846) radius 1.25
  circle A17 centre (-88, -9.8333) radius 1.25
  circle A18 centre (-88, -7.7821) radius 1.25
  circle A19 centre (-88, -5.7308) radius 1.25
  circle A20 centre (-88, -3.6795) radius 1.25
  circle A21 centre (-88, -1.6282) radius 1.25
  circle A22 centre (-88, 0.4231) radius 1.25
  circle A23 centre (-88, 2.4744) radius 1.25
  circle A24 centre (-88, 4.5256) radius 1.25
  circle A25 centre (-88, 6.5769) radius 1.25
  circle A26 centre (-88, 8.6282) radius 1.25
  circle A27 centre (-88, 10.6795) radius 1.25
  circle A28 centre (-88, 12.7308) radius 1.25
  circle A29 centre (-88, 14.7821) radius 1.25
  circle A30 centre (-88, 16.8333) radius 1.25
  circle A31 centre (-88, 18.8846) radius 1.25
  circle A32 centre (-88, 20.9359) radius 1.25
  circle A33 centre (-88, 22.9872) radius 1.25
  circle A34 centre (-88, 25.0385) radius 1.25
  circle A35 centre (-88, 27.0897) radius 1.25
  circle A36 centre (-88, 29.141) radius 1.25
  circle A37 centre (-88, 31.1923) radius 1.25
  circle A38 centre (-88, 33.2436) radius 1.25
  circle A39 centre (-88, 35.2949) radius 1.25
  circle A40 centre (-88, 37.3462) radius 1.25
  circle A41 centre (-88, 39.3974) radius 1.25
  circle A42 centre (-88, 41.4487) radius 1.25
  circle A43 centre (-88, 43.5) radius 1.25
  dimension "d170" = 4
  dimension "d171" = 2.5
  dimension "d172" = 40
  dimension "d175" = 0
  dimension "d176" = 80
  constraint concentric A1 A2
  constraint concentric A0 A3
  constraint equal A2 A3
  constraint coincident L0 A4.centre
  measures "d170" diameter of A2
  measures "d171" diameter of A4
  measures "d172" distance of A4.centre L6
extrude "Extrusion22" cut sketch "Skizze3" against normal blind 8 contours L0 L5 A1 A2 | L0 L5 A1 A2 | L0 A4 A5 | L0 A4 A5 | L0 A4 A5 | L0 A4 A5 | L0 A4 A5 A6 | L0 A4 A5 A6 | L0 A5 A6 A7 | L0 A5 A6 | L0 A5 A6 | L0 A5 A6 A7 | L0 A6 A7 A8 | L0 A6 A7 | L0 A6 A7 | L0 A6 A7 A8 | L0 A7 A8 A9 | L0 A7 A8 | L0 L6 A23 | L0 A23 A24 A25 | L0 A22 A23 A24 | L0 L6 A24 | L0 A7 A8 | L0 A7 A8 A9 | L0 A8 A9 A10 | L0 A8 A9 | L0 L6 A24 | L0 L6 A23 | L0 A23 A24 A25 | L0 A21 A22 A23 | L0 A22 A23 | L0 A24 A25 A26 | L0 A24 A25 | L0 A22 A23 A24 | L0 A8 A9 | L0 A8 A9 A10 | L0 A9 A10 A11 | L0 A9 A10 | L0 A0 L1 A3 | L0 A0 L1 A3 | L0 A24 A25 | L0 A22 A23 | L0 A20 A21 A22 | L0 A21 A22 | L0 A21 A22 A23 | L0 A24 A25 A26 | L0 A25 A26 A27 | L0 A25 A26 | L0 A9 A10 | L0 A9 A10 A11 | L0 A10 A11 A12 | L0 A10 A11 | L0 A21 A22 | L0 A19 A20 A21 | L0 A20 A21 | L0 A20 A21 A22 | L0 A25 A26 | L0 A25 A26 A27 | L0 A26 A27 A28 | L0 A26 A27 | L0 A10 A11 | L0 A10 A11 A12 | L0 A11 A12 A13 | L0 A11 A12 | L0 A42 A43 | L0 A42 A43 | L0 A20 A21 | L0 A18 A19 A20 | L0 A19 A20 | L0 A19 A20 A21 | L0 A26 A27 | L0 A26 A27 A28 | L0 A27 A28 A29 | L0 A27 A28 | L0 A11 A12 | L0 A11 A12 A13 | L0 A12 A13 A14 | L0 A12 A13 | L0 A42 A43 | L0 A42 A43 | L0 A41 A42 A43 | L0 A19 A20 | L0 A17 A18 A19 | L0 A18 A19 | L0 A18 A19 A20 | L0 A27 A28 | L0 A27 A28 A29 | L0 A28 A29 A30 | L0 A28 A29 | L0 A12 A13 | L0 A12 A13 A14 | L0 A13 A14 A15 | L0 A13 A14 | L0 A41 A42 A43 | L0 A40 A41 A42 | L0 A41 A42 | L0 A18 A19 | L0 A16 A17 A18 | L0 A17 A18 | L0 A17 A18 A19 | L0 A28 A29 | L0 A28 A29 A30 | L0 A29 A30 A31 | L0 A29 A30 | L0 A13 A14 | L0 A13 A14 A15 | L0 A14 A15 A16 | L0 A14 A15 | L0 A41 A42 | L0 A39 A40 A41 | L0 A40 A41 | L0 A40 A41 A42 | L0 A17 A18 | L0 A15 A16 A17 | L0 A16 A17 | L0 A16 A17 A18 | L0 A29 A30 | L0 A29 A30 A31 | L0 A30 A31 A32 | L0 A30 A31 | L0 A14 A15 | L0 A14 A15 A16 | L0 A15 A16 | L0 A40 A41 | L0 A38 A39 A40 | L0 A39 A40 | L0 A39 A40 A41 | L0 A16 A17 | L0 A15 A16 A17 | L0 A30 A31 | L0 A30 A31 A32 | L0 A31 A32 A33 | L0 A31 A32 | L0 A15 A16 | L0 A39 A40 | L0 A37 A38 A39 | L0 A38 A39 | L0 A38 A39 A40 | L0 A31 A32 | L0 A31 A32 A33 | L0 A32 A33 A34 | L0 A32 A33 | L0 A38 A39 | L0 A36 A37 A38 | L0 A37 A38 | L0 A37 A38 A39 | L0 A32 A33 | L0 A32 A33 A34 | L0 A33 A34 A35 | L0 A33 A34 | L0 A37 A38 | L0 A35 A36 A37 | L0 A36 A37 | L0 A36 A37 A38 | L0 A33 A34 | L0 A33 A34 A35 | L0 A34 A35 A36 | L0 A34 A35 | L0 A36 A37 | L0 A35 A36 | L0 A35 A36 A37 | L0 A34 A35 | L0 A34 A35 A36 | L0 A35 A36 bodies 11
extrude "Extrusion18" add sketch "Skizze1" along normal blind 16 and the other way blind -12 contours L3 L93 L94 L95 A32 L107 | L7 L93 L100 L101 A32 | L7 L93 L96 L97 L98 L99 A31 | L3 L92 L93 L95 L99 A31 L106 | L8 L84 L90 L91 | L8 L17 L68 L84 | L8 L84 L86 L87 L88 L89 | L8 L19 L70 L84 | L2 L17 L67 L68 L82 L84 | L2 L19 L67 L70 L82 L84 | A27 | A28 | A29 | A30 bodies 10 11
extrude "Extrusion20" cut sketch "Skizze1" along normal blind 6 and the other way blind -5 contours L41 L46 L104 L105 | L43 L48 L102 L103 bodies 6
extrude "Extrusion21" cut sketch "Skizze1" along normal blind 19 and the other way blind -17 contours L41 L46 L104 L105 | L43 L48 L102 L103 bodies 6
chamfer "Fase7" distance 1.5 angle 45 2 edges at (10.5, 59.5, 6) (10.5, 26.5, 6) on bodies 6
chamfer "Fase8" distance 1 angle 45 2 edges at (10.5, 28, 5) (10.5, 58, 5) on bodies 6
chamfer "Fase9" distance 1 angle 45 2 edges at (10.5, 59.5, 17) (10.5, 26.5, 17) on bodies 6
fillet "Abrundung5" radius 2 6 edges at (-25, 66, 11) (-25, 52.5, 11) (-15, 66, 11) (38, 66, 11) (48, 66, 11) (48, 52.5, 11) on bodies 6
named bodies: "frame", "display_backplate", "ESP_box", "display_cable_box", "long_grid", "short_grid"
